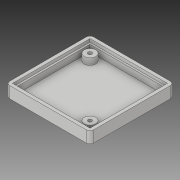
# Autodesk Inventor part: elec_detect_bucket
Saved by Autodesk Inventor 2019 (Build 230136000, 136)
## iProperties
Created: 2019-10-24
Part Number: elec_detect_bucket
Material: Generic
Document SubType Name: Modeling
Designer: devon
Density: 1 g/cm^3
Appearance: Default
Author: devon
Autodesk Inventor part; units mm, degrees
ref_plane "YZ Plane" through (0, 0, 0) normal (1, 0, 0) x (0, 1, 0)
ref_plane "XZ Plane" through (0, 0, 0) normal (0, 1, 0) x (-1, 0, 0)
ref_plane "XY Plane" through (0, 0, 0) normal (0, 0, 1) x (1, 0, 0)
sketch "Sketch1" plane through (0, 0, 0) normal (0, 1, 0) x (-1, 0, 0)
  line L0 (22, 22) -> (-22, 22)
  line L1 (-22, 22) -> (-22, -22)
  line L2 (-22, -22) -> (22, -22)
  line L3 (22, -22) -> (22, 22)
  line L4 (22, 22) -> (-22, -22) construction
  line L5 (-22, 22) -> (22, -22) construction
  point P0 (0, 0)
  dimension "d0" = 44
  dimension "d1" = 44
  constraints: 12 end point, 2 midpoint, 2 parallel, 1 horizontal, 1 perpendicular
  measures "d0" distance of L1.end L2.end
  measures "d1" distance of L2.end L0.start
extrude "Extrusion1" add sketch "Sketch1" along normal blind 6
sketch "Sketch2" plane through (0, 6, 0) normal (0, 1, 0) x (1, 0, 0)
  line L0 (-20.3, -20.3) -> (20.3, -20.3)
  line L1 (20.3, -20.3) -> (20.3, 20.3)
  line L2 (20.3, 20.3) -> (-20.3, 20.3)
  line L3 (-20.3, 20.3) -> (-20.3, -20.3)
  line L4 (-20.3, -20.3) -> (20.3, 20.3) construction
  line L5 (20.3, -20.3) -> (-20.3, 20.3) construction
  point P0 (0, 0)
  dimension "d4" = 40.6
  dimension "d5" = 40.6
  constraints: 12 end point, 2 midpoint, 2 parallel, 1 horizontal, 1 perpendicular
  measures "d4" distance of L1.end L2.end
  measures "d5" distance of L2.end L0.start
extrude "Extrusion2" cut sketch "Sketch2" against normal blind 1.6
sketch "Sketch3" plane through (0, 4.4, 0) normal (0, 1, 0) x (1, 0, 0)
  line L0 (-19.3, -19.3) -> (19.3, -19.3)
  line L1 (19.3, -19.3) -> (19.3, 19.3)
  line L2 (19.3, 19.3) -> (-19.3, 19.3)
  line L3 (-19.3, 19.3) -> (-19.3, -19.3)
  line L4 (-19.3, -19.3) -> (19.3, 19.3) construction
  line L5 (19.3, -19.3) -> (-19.3, 19.3) construction
  point P0 (0, 0)
  dimension "d8" = 38.6
  dimension "d9" = 38.6
  constraints: 12 end point, 2 midpoint, 2 parallel, 1 horizontal, 1 perpendicular
  measures "d8" distance of L1.end L2.end
  measures "d9" distance of L2.end L0.start
extrude "Extrusion3" cut sketch "Sketch3" against normal blind 3.4
sketch "Sketch4" plane through (0, 1, 0) normal (0, 1, 0) x (1, 0, 0)
  circle A0 centre (-15.3, 15.3) radius 3
  circle A1 centre (15.3, -15.3) radius 3
  line L0 (-20.3, 20.3) -> (20.3, 20.3) projected
  line L1 (-20.3, -20.3) -> (-20.3, 20.3) projected
  line L2 (20.3, 20.3) -> (20.3, -20.3) projected
  line L3 (20.3, -20.3) -> (-20.3, -20.3) projected
  point P0 (0, 0)
  dimension "d12" = 5
  dimension "d13" = 5
  dimension "d14" = 6
  dimension "d15" = 5
  dimension "d16" = 5
  dimension "d17" = 6
  constraints: 2 centre point
  measures "d12" distance from line of L0 A0.centre
  measures "d13" distance from line of L1 A0.centre
  measures "d14" diameter of A0
  measures "d15" distance from line of L2 A1.centre
  measures "d16" distance from line of L3 A1.centre
  measures "d17" diameter of A1
extrude "Extrusion4" add sketch "Sketch4" along normal blind 3.4 contours A0 | A1
sketch "Sketch5" plane through (-15.3, 4.4, -15.3) normal (0, 1, 0) x (1, 0, 0)
  circle A0 centre (0, 0) radius 1
  circle A1 centre (30.6, -30.6) radius 3 projected
  circle A2 centre (30.6, -30.6) radius 1
  point P0 (15.3, -15.3)
  dimension "d20" = 2
  dimension "d21" = 2
  constraints: 2 centre point, 1 coincident
  measures "d20" diameter of A0
  measures "d21" diameter of A2
extrude "Extrusion5" cut sketch "Sketch5" against normal blind 3.4 contours A0 | A2
fillet "Fillet1" radius 2 4 edges at (-22, 3, -22) (22, 3, -22) (22, 3, 22) (-22, 3, 22)
body "Solid1"
